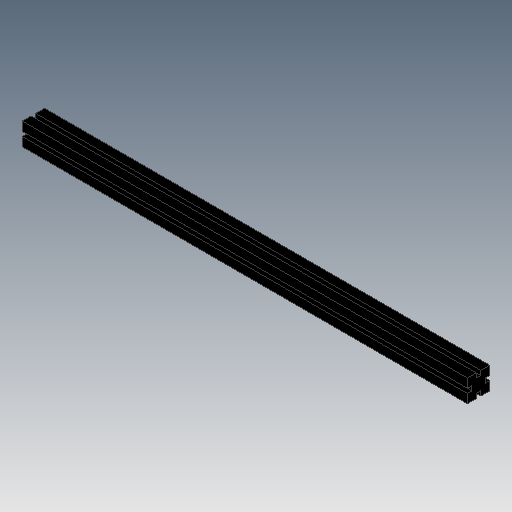
# Autodesk Inventor part: Beam_300mm
Saved by Autodesk Inventor 2018.3 (Build 223284000, 284)
## iProperties
Created: 2020-05-08
Part Number: Beam_300mm
Material: Aluminum 6061
Document SubType Name: Modeling
Designer: Remo
Mass: 153.09 g
Surface Area: 255.78 cm^2
Volume: 56.7 cm^3
Density: 2.7 g/cm^3
Appearance: Anodized - Black
Description: OpenBeam 300mm 15x15 Aluminium Beam
Author: Remo
Autodesk Inventor part; units mm, degrees
ref_plane "YZ Plane" through (0, 0, 0) normal (1, 0, 0) x (0, 1, 0)
ref_plane "XZ Plane" through (0, 0, 0) normal (0, 1, 0) x (-1, 0, 0)
ref_plane "XY Plane" through (0, 0, 0) normal (0, 0, 1) x (1, 0, 0)
sketch "Sketch1" plane through (0, 0, 0) normal (1, 0, 0) x (0, 1, 0)
  line L0 (-7.5, -7.5) -> (7.5, -7.5)
  line L1 (7.5, -7.5) -> (7.5, 7.5)
  line L2 (7.5, 7.5) -> (-7.5, 7.5)
  line L3 (-7.5, 7.5) -> (-7.5, -7.5)
  line L4 (-7.5, -7.5) -> (7.5, 7.5) construction
  line L5 (7.5, -7.5) -> (-7.5, 7.5) construction
  line L6 (7.5, 1.5) -> (4.5, 1.5)
  line L7 (4.5, 1.5) -> (4.5, -1.5)
  line L8 (4.5, -1.5) -> (7.5, -1.5)
  line L9 (7.5, -1.5) -> (7.5, 1.5)
  line L10 (1.5, 7.5) -> (-1.5, 7.5)
  line L11 (-1.5, 7.5) -> (-1.5, 4.5)
  line L12 (-1.5, 4.5) -> (1.5, 4.5)
  line L13 (1.5, 4.5) -> (1.5, 7.5)
  line L14 (-7.5, 1.5) -> (-4.5, 1.5)
  line L15 (-4.5, 1.5) -> (-4.5, -1.5)
  line L16 (-4.5, -1.5) -> (-7.5, -1.5)
  line L17 (-7.5, -1.5) -> (-7.5, 1.5)
  line L18 (-1.5, -7.5) -> (1.5, -7.5)
  line L19 (1.5, -7.5) -> (1.5, -4.5)
  line L20 (1.5, -4.5) -> (-1.5, -4.5)
  line L21 (-1.5, -4.5) -> (-1.5, -7.5)
  point P0 (0, 0)
  dimension "d0" = 15
  dimension "d1" = 3
  dimension "d2" = 3
  dimension "d3" = 1.5
  dimension "d4" = 1.5
  constraints: 44 end point, 10 parallel, 10 perpendicular, 5 horizontal, 4 point on line, 2 horizontal alignment, 2 midpoint, 2 vertical alignment
  measures "d0" distance of L0.end L1.end
  measures "d1" distance of L7.end L8.end
  measures "d2" distance of L6.end L7.end
  measures "d3" distance from line of point (0, 0) L8
  measures "d4" distance from line of point (0, 0) L19
extrude "Extrusion1" add sketch "Sketch1" along normal blind 300 contours L3 L16 L15 L14 L2 L11 L12 L13 L1 L6 L7 L8 L0 L19 L20 L21
equation "\"d3\" = 0.5 * d2"
equation "\"d4\" = d3"
body "Solid1"
